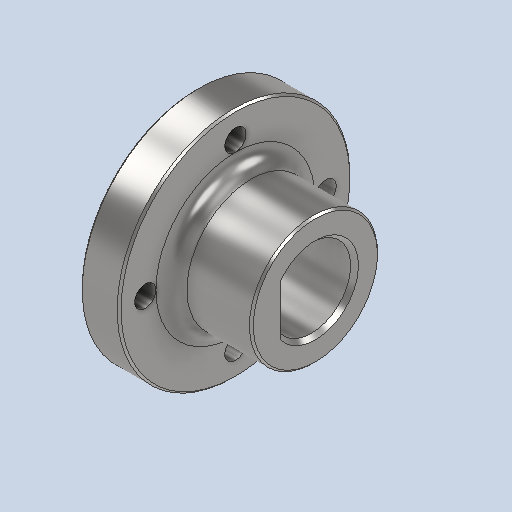
# Autodesk Inventor part: Flansch_Wellennabeverbindung_MainAxis
Saved by Autodesk Inventor 2022 (Build 260153000, 153)
## iProperties
Created: 2022-07-14
Part Number: Flansch_Wellennabeverbindung_MainAxis
Material: Edelstahl
Document SubType Name: Modeling
Designer: alexw
Density: 8 g/cm^3
Appearance: Halbpoliert
Mass: 271.614 g
Surface Area: 119.643 cm^2
Volume: 33.9518 cm^3
Flansch_Klemmdeckelausnahme_Dia: 27,000 mm
Flansch_Rad: 10,000 mm
Flansch_MalePart_Height: 2,200 mm
Flansch_FemalePart_OuterDia: 30,000 mm
Flansch_Number_Holes: 4,000 oE
Flansch_FemalePart_HoleDia: 46,500 mm
Author: alexw
Autodesk Inventor part; units mm, degrees
ref_plane "YZ Plane" through (0, 0, 0) normal (1, 0, 0) x (0, 1, 0)
ref_plane "XZ Plane" through (0, 0, 0) normal (0, 1, 0) x (-1, 0, 0)
sketch "Skizze1" plane through (0, 0, 0) normal (0, 0, 1) x (1, 0, 0)
  line L0 (0, 13.5) -> (0, 30)
  line L1 (0, 30) -> (10, 30)
  line L2 (10, 30) -> (10, 16.5)
  line L3 (10, 16.5) -> (30.6, 16.5)
  line L4 (30.6, 16.5) -> (30.6, 10)
  line L5 (30.6, 10) -> (5, 10)
  line L6 (-6.12, 0) -> (36.72, 0) construction
  line L7 (0, -6) -> (0, 36) construction
  line L8 (0, 13.5) -> (5, 13.5)
  line L9 (5, 13.5) -> (5, 10)
  line L10 (5, 12.8) -> (30.6, 12.8) construction
  line L11 (10, 16.5) -> (10, 0) construction
  line L12 (2.2, 13.5) -> (2.2, 0) construction
  point P0 (0, 0)
  dimension "d0" = 10
  dimension "d1" = 25.6
  dimension "d2" = 2.8
  dimension "Flansch_FemalePart_OuterDia" = 30
  dimension "d13" = 0.7
  dimension "Flansch_Klemmdeckelausnahme_Dia" = 27
  dimension "d36" = 10
  dimension "d37" = 5
  dimension "d38" = 2.8
  dimension "Flansch_MalePart_Height" = 2.2
  dimension "d40" = 33
  constraints: 22 end point, 7 perpendicular, 6 point on line, 2 vertical, 1 parallel, 2 other
  measures "d0" distance between parallel lines of L5 L6
  measures "d1" distance between parallel lines of L4 L9
  measures "d2" distance between parallel lines of L10 L5
  measures "Flansch_FemalePart_OuterDia" distance between parallel lines of L1 L6
  measures "d13" distance between parallel lines of L10 L8
  measures "Flansch_Klemmdeckelausnahme_Dia" diameter of L8 L6
  measures "d36" distance of L0.end L1.end
  measures "d37" distance between parallel lines of L11 L9
  measures "d38" distance between parallel lines of L9 L12
  measures "Flansch_MalePart_Height" distance of the line from the sketch origin of L12
  measures "d40" diameter of L3 L6
revolve "Umdrehung1" add sketch "Skizze1" angle 360 about axis through (-10, 0, 0) along (1, 0, 0)
ref_plane "Nabennut_Arbeitsebene" through (17.8, 0, 10) normal (0, 0, 1) x (1, 0, 0)
sketch "Skizze2" plane through (17.8, 0, 10) normal (0, 0, 1) x (1, 0, 0)
  line L0 (-12.8, -13.5) -> (-12.8, 13.5) construction
  line L1 (12.8, -16.5) -> (12.8, 16.5) construction
  line L2 (-12.8, 3) -> (12.8, 3)
  line L3 (12.8, 3) -> (12.8, -3)
  line L4 (12.8, -3) -> (-12.8, -3)
  line L5 (-12.8, -3) -> (-12.8, 3)
  point P0 (-17.8, 0)
  point P1 (12.8, 0)
  dimension "d8" = 6
  constraints: 8 end point, 2 midpoint, 2 parallel, 2 point on line, 1 horizontal, 1 perpendicular
  measures "d8" distance between parallel lines of L4 L2
extrude "Extrusion1" cut sketch "Skizze2" along normal blind 2.8 and the other way blind 2
sketch "Skizze3" plane through (0, 0, 0) normal (-1, 0, 0) x (0, 0, 1)
  circle A0 centre (0, 0) radius 30 construction
  circle A1 centre (0, 0) radius 23.25 construction
  circle A2 centre (0, 0) radius 13.5 construction
  circle A3 centre (0, 0) radius 16.5 construction
  line L0 (0, 0) -> (23.25, 0) construction
  line L1 (0, 0) -> (16.5, 0) construction
  point P0 (0, 23.25)
  point P1 (-23.25, 0)
  point P2 (0, -23.25)
  dimension "d32" = 33
  dimension "Flansch_FemalePart_HoleDia" = 46.5
  dimension "d15" = 27
  dimension "d16" = 60
  dimension "d23" = 360
  dimension "d41" = 0
  constraints: 4 end point, 2 horizontal alignment, 1 coincident, 1 horizontal, 8 other
  measures "d15" diameter of A2
  measures "d16" diameter of A0
  measures "d41" distance between parallel lines of L0 L1
hole "Bohrung1" at (0, 0, 23.25) at (0, 23.25, 0) at (0, 0, -23.25) at (0, -23.25, 0) direction (1, 0, 0) diameter 5.5 end through all clearance for "Inbusschraube DIN EN ISO 4762" size "M5" standard "DIN"
sketch "Skizze4" plane through (30.6, 0, 0) normal (1, 0, 0) x (0, 0, -1)
  line L0 (-12.8, 3) -> (-9.5394, 3) projected
  line L1 (-12.8, -3) -> (-12.8, 3) projected
  line L2 (-9.5394, -3) -> (-12.8, -3) projected
  arc A0 (-9.5394, -3) -> (-9.5394, 3) centre (0, 0) ccw projected
  arc A1 (-9.5394, -3) -> (-9.5394, 3) centre (0, 0) ccw construction
  circle A2 centre (0, 0) radius 10
  line L3 (-8, 6) -> (-8, -6)
  line L4 (-10, 0) -> (0, 0) construction
  line L5 (0, 0) -> (0, -10) construction
  line L6 (8, 6) -> (8, -6)
  dimension "d19" = 45
  dimension "d43" = 2
  constraints: 8 end point, 5 point on circle, 2 symmetric about line, 2 vertical, 1 centre point, 1 coincident, 1 horizontal
  measures "d43" distance from line of L3 L4.start
extrude "Extrusion2" add sketch "Skizze4" against normal up to surface (25.6 mm away) contours L0 A2 L2 L1 | A0 L3 A2
thicken "Verdickung1" operation add thickness 0.1 both sides no extend neighbours yes toward (0, 0.971698, -0.2362267) faces at (22.0667, 9.717, -2.3623) (13.5333, -2, 8)
thicken "Verdickung2" operation add thickness 0.15 both sides no extend neighbours yes toward (0, -0.7865065, -0.6175819) faces at (3.3333, -10.6178, -8.3374)
chamfer "Fase2" distance 1 angle 45 2 edges at (30.6, 0, -10.1) (30.6, 0, 8.1)
chamfer "Fase1" distance 0.5 angle 45 6 edges at (0, -30, 0) (30.6, -16.5, 0) (10, -30, 0) (0, -13.65, 0) (5, 0, -10.1) (5, 0, 8.1)
fillet "Rundung1" radius 4 1 edges at (10, -16.5, 0)
equation "\"d0\" = Flansch_Rad"
equation "\"d2\" = Nabennuttiefe"
equation "\"d8\" = Passfeder_width"
equation "\"d9\" = Nabennuttiefe"
equation "\"Flansch_FemalePart_HoleDia\" = 0.5 * d16 + 0.5 * d32"
equation "\"Flansch_Rad\" = 10"
equation "\"Nabennuttiefe\" = 2.8"
equation "\"Passfeder_width\" = 6"
